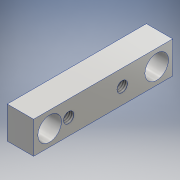
# Autodesk Inventor part: HeadbarHolderBracket_v2
Saved by Autodesk Inventor 2016 (Build 200138000, 138)
## iProperties
Created: 2015-11-11
Part Number: HeadbarHolderBracket_v2
Material: Aluminum 6061
Document SubType Name: Modeling
Designer: runeala
Mass: 43.2767 g
Surface Area: 66.3346 cm^2
Volume: 16.0284 cm^3
Density: 2.7 g/cm^3
Appearance: Aluminum - Flat
Author: runeala
Autodesk Inventor part; units mm, degrees
ref_plane "YZ Plane" through (0, 0, 0) normal (1, 0, 0) x (0, 1, 0)
ref_plane "XZ Plane" through (0, 0, 0) normal (0, 1, 0) x (-1, 0, 0)
ref_plane "XY Plane" through (0, 0, 0) normal (0, 0, 1) x (1, 0, 0)
sketch "Sketch1" plane through (0, 0, 0) normal (0, 1, 0) x (-1, 0, 0)
  line L0 (0, 0) -> (12.3, 0)
  line L1 (12.3, 0) -> (12.3, 15)
  line L2 (12.3, 15) -> (0, 15)
  line L3 (0, 15) -> (0, 0)
  dimension "d0" = 15
  dimension "d1" = 12.3
  constraints: 8 end point, 2 parallel, 1 horizontal, 1 perpendicular
  measures "d0" distance of L0.end L1.end
  measures "d1" distance of L1.end L2.end
extrude "Extrusion1" add sketch "Sketch1" along normal mid plane 65
sketch "Sketch2" plane through (-12.3, -32.5, 15) normal (-1, 0, 0) x (0, 0, 1)
  circle A0 centre (-7.5, 7.5) radius 3.25
  circle A1 centre (-7.5, 57.5) radius 3.25
  circle A2 centre (-7.5, 7.5) radius 5.5
  circle A3 centre (-7.5, 57.5) radius 5.5
  line L0 (0, 0) -> (-15, 0) projected
  line L1 (-15, 32.5) -> (12.3047, 32.5) construction
  dimension "d4" = 6.5
  dimension "d5" = 6.5
  dimension "d8" = 11
  dimension "d9" = 11
  dimension "d26" = 25
  dimension "d27" = 25
  constraints: 4 centre point, 2 coincident, 2 end point, 1 horizontal
  measures "d4" diameter of A0
  measures "d5" diameter of A1
  measures "d8" diameter of A2
  measures "d9" diameter of A3
  measures "d26" distance from line of L1 A1.centre
  measures "d27" distance from line of L1 A0.centre
extrude "Extrusion2" cut sketch "Sketch2" against normal through all contours A0 | A1
extrude "Extrusion3" cut sketch "Sketch2" against normal blind 21.3
sketch "Sketch3" plane through (-12.3, -32.5, 15) normal (-1, 0, 0) x (0, 0, 1)
  circle A0 centre (-7.5, 16.395) radius 3
  line L0 (0, 0) -> (-15, 0) projected
  circle A1 centre (-7.5, 41.395) radius 3
  point P0 (-15, 32.5)
  dimension "d14" = 6
  dimension "d22" = 16.395
  dimension "d23" = 6
  dimension "d24" = 25
  constraints: 2 centre point
  measures "d14" diameter of A0
  measures "d22" distance from line of L0 A0.centre
  measures "d23" diameter of A1
  measures "d24" distance of A0.centre A1.centre
hole "Hole1" at (-12.3, -16.105, 7.5) at (-12.3, 8.895, 7.5) direction (1, 0, 0) diameter 4.917 depth 15.1 tip angle 118 thread size "M6x1" class "6H" standard "ANSI Metric M Profile"
sketch "Sketch4" plane through (-12.3, -32.5, 15) normal (-1, 0, 0) x (0, 0, 1)
  point P0 (-15, 32.5)
body "Solid1"
